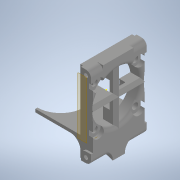
# Autodesk Inventor part: hotend_fan_mount
Saved by Autodesk Inventor 2022 (Build 260153000, 153)
## iProperties
Created: 2021-11-28
Part Number: hotend_fan_mount
Material: Polycarbonate, Clear
Document SubType Name: Modeling
Designer: alexr
Density: 1.2 g/cm^3
Appearance: Polycarbonate - Clear
Mass: 4.68895 g
Surface Area: 35.8129 cm^2
Volume: 3.90746 cm^3
Author: alexr
Autodesk Inventor part; units mm, degrees
ref_plane "YZ Plane" through (0, 0, 0) normal (1, 0, 0) x (0, 1, 0)
ref_plane "XZ Plane" through (0, 0, 0) normal (0, 1, 0) x (-1, 0, 0)
ref_plane "XY Plane" through (0, 0, 0) normal (0, 0, 1) x (1, 0, 0)
sketch "Sketch1" plane through (0, 0, 0) normal (1, 0, 0) x (0, 1, 0)
  line L0 (-12.75, -12.75) -> (12.75, -12.75)
  line L1 (12.75, -12.75) -> (12.75, 12.75)
  line L2 (12.75, 12.75) -> (-12.75, 12.75)
  line L3 (-12.75, 12.75) -> (-12.75, -12.75)
  line L4 (-12.75, -12.75) -> (12.75, 12.75) construction
  line L5 (12.75, -12.75) -> (-12.75, 12.75) construction
  circle A0 centre (0, 0) radius 12
  circle A1 centre (10, 10) radius 1.5
  circle A2 centre (10, -10) radius 1.5
  circle A3 centre (-10, 10) radius 1.5
  circle A4 centre (-10, -10) radius 1.5
  line L6 (-12.2199, 1.5) -> (12.2199, 1.5)
  line L7 (12.2199, 1.5) -> (12.2199, -1.5)
  line L8 (12.2199, -1.5) -> (-12.2199, -1.5)
  line L9 (-12.2199, -1.5) -> (-12.2199, 1.5)
  line L10 (-12.2199, 1.5) -> (12.2199, -1.5) construction
  line L11 (12.2199, 1.5) -> (-12.2199, -1.5) construction
  line L12 (-1.5, -12.2199) -> (1.5, -12.2199)
  line L13 (1.5, -12.2199) -> (1.5, 12.2199)
  line L14 (1.5, 12.2199) -> (-1.5, 12.2199)
  line L15 (-1.5, 12.2199) -> (-1.5, -12.2199)
  line L16 (-1.5, -12.2199) -> (1.5, 12.2199) construction
  line L17 (1.5, -12.2199) -> (-1.5, 12.2199) construction
  point P0 (1.5, -1.5)
  point P1 (11.9059, -1.5)
  point P2 (11.9059, 1.5)
  point P3 (1.5, 1.5)
  point P4 (1.5, 11.9059)
  point P5 (-1.5, 11.9059)
  point P6 (-1.5, 1.5)
  point P7 (-11.9059, 1.5)
  point P8 (-11.9059, -1.5)
  point P9 (-1.5, -1.5)
  point P10 (-1.5, -11.9059)
  point P11 (1.5, -11.9059)
  dimension "d0" = 25.5
  dimension "d1" = 25.5
  dimension "d2" = 24
  dimension "d3" = 3
  dimension "d4" = 3
  dimension "d5" = 20
  dimension "d6" = 2.75
  dimension "d7" = 3
  dimension "d8" = 3
  dimension "d11" = 3
  dimension "d12" = 3
  constraints: 36 end point, 6 midpoint, 6 parallel, 5 centre point, 4 point on line, 3 horizontal, 3 perpendicular, 1 coincident
  measures "d0" distance of L2.end L1.end
  measures "d1" distance of L1.end L0.end
  measures "d2" diameter of A0
  measures "d3" diameter of A1
  measures "d4" diameter of A2
  measures "d5" distance of A2.centre A1.centre
  measures "d6" distance from line of L2 A1.centre
  measures "d7" diameter of A3
  measures "d8" diameter of A4
  measures "d11" distance of L6.end L7.end
  measures "d12" distance of L14.end L13.end
extrude "Extrusion1" add sketch "Sketch1" along normal blind 6.25 contours L3 L2 L1 L0 | A0 L8 L13 L6 | A0 L6 L7 L8 | L13 L6 L15 A0 | A0 L15 L14 L13 | L13 L8 L15 L6 | L13 L12 L15 A0 | A0 L15 L8 L13 | L15 L8 A0 L6 | A0 L8 L9 L6
ref_plane "Work Plane1" through (0, -12.75, 13.75) normal (0, 0, 1) x (1, 0, 0)
sketch "Sketch2" plane through (0, -12.75, 13.75) normal (0, 0, 1) x (1, 0, 0)
  arc A0 (6.25, 27.5) -> (3.75, 30) centre (3.75, 27.5) ccw projected
  line L0 (6.25, 27.5) -> (6.25, 25) projected
  line L1 (3.7511, 25) -> (6.25, 25) projected
  arc A1 (1.25, 27.5011) -> (3.7511, 25) centre (3.75, 27.5) ccw projected
  line L2 (1.25, 30) -> (1.25, 27.5011) projected
  line L3 (1.25, 30) -> (3.75, 30) projected
  circle A2 centre (3.75, 27.5) radius 1 projected
  arc A3 (3.75, -10) -> (6.25, -7.5) centre (3.75, -7.5) ccw projected
  line L4 (3.75, -10) -> (1.25, -10) projected
  line L5 (1.25, -7.5011) -> (1.25, -10) projected
  arc A4 (3.7511, -5) -> (1.25, -7.5011) centre (3.75, -7.5) ccw projected
  line L6 (6.25, -5) -> (3.7511, -5) projected
  line L7 (6.25, -5) -> (6.25, -7.5) projected
  circle A5 centre (3.75, -7.5) radius 1 projected
  point P0 (0, 12.75)
extrude "Extrusion2" add sketch "Sketch2" against normal blind 14.5
sketch "Sketch3" plane through (0, 12.75, 12.75) normal (0, 1, 0) x (1, 0, 0)
  line L0 (-19.75, 12.3932) -> (-19.75, 3.5868) projected
  line L1 (0, 0) -> (6.25, 0) projected
  line L2 (2.25, 13.5) -> (6.25, 13.5) projected
  line L3 (0, 0) -> (2.3102, 0)
  line L4 (2.3102, 0) -> (2.3102, 13.5)
  line L5 (2.3102, 13.5) -> (0, 13.5)
  line L6 (0, 13.5) -> (0, 0)
  point P0 (0, 12.75)
  constraints: 8 end point, 2 parallel, 1 horizontal, 1 perpendicular, 1 point on line
extrude "Extrusion3" add sketch "Sketch3" along normal blind 4.5
sketch "Sketch4" plane through (0, 0, 0) normal (-1, 0, 0) x (0, 0, 1)
  point P0 (0, 0)
sketch "Sketch5" plane through (0, -12.75, 12.75) normal (0, 0, 1) x (1, 0, 0)
  line L0 (0, 0) -> (6.25, 0) projected
  line L1 (0, 0) -> (0, -10)
  line L2 (1.25, -10) -> (3.75, -10) projected
  line L3 (0, -10) -> (1.25, -10)
  line L4 (6.25, 0) -> (6.25, -5)
  arc A0 (3.7511, -5) -> (1.25, -7.5011) centre (3.75, -7.5) ccw projected
  line L5 (6.25, -5) -> (3.7511, -5) projected
  line L6 (1.25, -7.5011) -> (1.25, -10) projected
  line L7 (6.25, -5) -> (3.7511, -5) projected
  line L8 (6.25, -5) -> (6.25, -5)
  line L9 (6.25, -5) -> (6.25, -5) construction
  point P0 (0, 12.75)
  dimension "d20" = 135
  constraints: 10 end point, 2 perpendicular, 1 equal length, 1 horizontal, 1 point on line, 1 vertical
  measures "d20" angle of L9 L8
extrude "Extrusion4" add sketch "Sketch5" against normal blind 14.5
mirror "Mirror2" about plane through (0, 0, 0) normal (0, 0, 1) of "Extrusion2", "Extrusion3", "Extrusion4"
sketch "Sketch6" plane through (6.25, 0, 0) normal (1, 0, 0) x (0, 0, -1)
  line L0 (13.75, 13.75) -> (-13.75, 13.75)
  line L1 (-7.75, 23.55) -> (-7.75, 17.35) projected
  line L2 (-7.75, 17.35) -> (7.25, 17.35) projected
  line L3 (13.75, 13.75) -> (-13.75, 13.75) projected
  line L4 (-7.75, 17.35) -> (7.25, 17.35)
  line L5 (7.25, 17.35) -> (7.25, 13.75)
  line L6 (7.25, 13.75) -> (-7.75, 13.75)
  line L7 (-7.75, 13.75) -> (-7.75, 17.35)
  line L8 (11.25, 23.55) -> (11.25, 17.35) projected
  line L9 (13.75, 13.75) -> (-13.75, 13.75) projected
  line L10 (7.25, 17.35) -> (11.25, 17.35)
  line L11 (11.25, 17.35) -> (11.25, 13.75)
  line L12 (11.25, 13.75) -> (7.25, 13.75)
  line L13 (7.25, 13.75) -> (7.25, 17.35)
  line L14 (-7.75, 23.55) -> (7.25, 23.55) projected
  line L15 (7.25, 17.35) -> (7.25, 23.55) projected
  point P0 (0, 0)
  point P1 (-7.75, 13.75)
  point P2 (7.25, 17.35)
  constraints: 18 end point, 4 parallel, 2 horizontal, 2 perpendicular, 2 point on line
extrude "Extrusion5" add sketch "Sketch6" against normal blind 3 contours L0 L7 L2 L5
sketch "Sketch7" plane through (3.75, 17.25, -13.75) normal (0, 0, -1) x (-1, 0, 0)
  circle A0 centre (0, -2.5) radius 1 projected
  point P0 (3.75, -17.25)
extrude "Extrusion6" cut sketch "Sketch7" against normal blind 30
sketch "Sketch8" plane through (6.25, 0, 0) normal (1, 0, 0) x (0, 0, -1)
  circle A0 centre (-10, 10) radius 2.85 projected
  circle A1 centre (-10, 10) radius 3
  circle A2 centre (10, 10) radius 1.45 projected
  circle A3 centre (-10, -10) radius 1.45 projected
  circle A4 centre (10, -10) radius 1.45 projected
  circle A5 centre (-10, -10) radius 3
  circle A6 centre (10, -10) radius 3
  circle A7 centre (10, 10) radius 3
  point P0 (0, 0)
  dimension "d25" = 6
  dimension "d26" = 6
  dimension "d27" = 6
  dimension "d28" = 6
  constraints: 4 centre point, 4 coincident
  measures "d25" diameter of A1
  measures "d26" diameter of A5
  measures "d27" diameter of A6
  measures "d28" diameter of A7
extrude "Extrusion7" cut sketch "Sketch8" against normal blind 2 contours A0 | A1 | A2 | A3 | A4 | A5 | A6 | A7
sketch "Sketch9" plane through (1.25, -22.75, 13.75) normal (0, -1, 0) x (1, 0, 0)
  line L0 (5, -15.25) -> (5, -20.7614) projected
  line L1 (-7.5, -10.75) -> (5, -10.75)
  line L2 (5, -10.75) -> (5, -16.75)
  line L3 (5, -16.75) -> (-7.5, -16.75)
  line L4 (-7.5, -16.75) -> (-7.5, -10.75)
  line L5 (-7.5, -10.75) -> (5, -16.75) construction
  line L6 (5, -10.75) -> (-7.5, -16.75) construction
  line L7 (-1.25, -1) -> (-1.25, -26.5) projected
  point P0 (-1.25, -13.75)
  point P1 (-1.25, -10.75)
  point P2 (-1.25, -16.75)
  dimension "d31" = 6
  constraints: 12 end point, 2 midpoint, 2 parallel, 1 horizontal, 1 perpendicular, 1 point on line
  measures "d31" distance of L1.end L2.end
extrude "Extrusion8" add sketch "Sketch9" along normal mid plane 6 contours L0 L3 L7 L1 L2
chamfer "Chamfer1" distance 6 distance2 3 1 edges at (0, -25.75, 0) measured on face at (0.5, -25.75, 0)
fillet "Fillet1" radius 3 4 edges at (1.875, -22.75, -3) (5.5178, -22.0178, -3) (1.875, -22.75, 3) (5.5178, -22.0178, 3)
fillet "Fillet2" radius 2 8 edges at (6.25, 4.3915, 11.1676) (6.25, 11.1676, 4.3915) (6.25, 11.1676, -4.3915) (6.25, 4.3915, -11.1676) (6.25, -4.3915, -11.1676) (6.25, -11.1676, -4.3915) (6.25, -11.1676, 4.3915) (6.25, -4.3915, 11.1676)
chamfer "Chamfer2" distance 1.45 angle 45 8 edges at (6.25, -1.5, 7.125) (6.25, 1.5, 7.125) (6.25, 7.7097, 1.5) (6.25, 7.7097, -1.5) (6.25, 1.5, -7.125) (6.25, -1.5, -7.125) (6.25, -7.7097, -1.5) (6.25, -7.7097, 1.5)
ref_plane "Work Plane2" through (0, -13, 1.5) normal (0, -1, 0) x (1, 0, 0)
sketch "Sketch10" plane through (0, -13, 1.5) normal (0, -1, 0) x (1, 0, 0)
  circle A0 centre (-22.25, -1.25) radius 11.175 projected
  line L0 (-28.75, 11.25) -> (1.25, 11.25) projected
  line L1 (1.25, -14.25) -> (-28.75, -14.25) projected
  circle A1 centre (-22.25, -1.25) radius 11.425
  line L2 (-22.25, -14.25) -> (-22.25, 11.25)
  line L3 (0, -14.25) -> (0, 11.25)
  point P0 (0, -1.5)
  point P1 (-22.25, 10.175)
  point P2 (-22.25, -12.675)
  dimension "d43" = 0.25
  constraints: 4 end point, 2 point on line, 1 centre point, 1 perpendicular
  measures "d43" radial gap between concentric circles of A0 A1
extrude "Extrusion9" add sketch "Sketch10" along normal blind 1.5 contours L2 L0 L3 L1 A1
fillet "Fillet3" radius 5 1 edges at (0, -14.5, 0)
sketch "Sketch11" plane through (0, 0, 0) normal (-1, 0, 0) x (0, 0, 1)
  circle A0 centre (0, 0) radius 6.5
  dimension "d47" = 13
  constraints: 1 centre point, 1 coincident
  measures "d47" diameter of A0
extrude "Extrusion10" cut sketch "Sketch11" against normal blind 3.175
equation "\"d1\" = d0"
equation "\"d6\" = -0.5 * d5 + 0.5 * d1"
body "Solid1"
